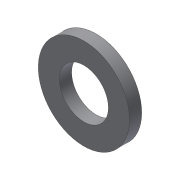
# Autodesk Inventor part: 90945A713_NAS620C5_flat_washer
Saved by Autodesk Inventor 2014 SP1 (Build 180222100, 222)
## iProperties
Created: 2019-06-26
Part Number: 90945A713_NAS620C5_flat_washer
Material: Generic
Document SubType Name: Modeling
Designer: RDavis
Density: 1 g/cm^3
Appearance: Default
Author: RDavis
Autodesk Inventor part; units mm, degrees
ref_plane "YZ Plane" through (0, 0, 0) normal (1, 0, 0) x (0, 1, 0)
ref_plane "XZ Plane" through (0, 0, 0) normal (0, 1, 0) x (-1, 0, 0)
ref_plane "XY Plane" through (0, 0, 0) normal (0, 0, 1) x (1, 0, 0)
sketch "Sketch1" plane through (0, 0, 0) normal (0, 0, 1) x (1, 0, 0)
  circle A0 centre (0, 0) radius 1.6256
  circle A1 centre (0, 0) radius 3.0226
  dimension "d0" = 3.2512
  dimension "d1" = 6.0452
  constraints: 2 centre point, 2 coincident
  measures "d0" diameter of A0
  measures "d1" diameter of A1
extrude "Extrusion1" add sketch "Sketch1" along normal mid plane 0.8128
body "Solid1"
